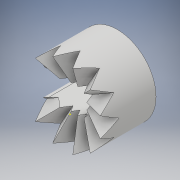
# Autodesk Inventor part: spodek
Saved by Autodesk Inventor 2018 (Build 220112000, 112)
## iProperties
Created: 2017-05-11
Part Number: spodek
Material: Všeobecné
Document SubType Name: Modeling
Designer: tonarr
Density: 1 g/cm^3
Appearance: Výchozí
Author: tonarr
Autodesk Inventor part; units mm, degrees
ref_plane "YZ Plane" through (0, 0, 0) normal (1, 0, 0) x (0, 1, 0)
ref_plane "XZ Plane" through (0, 0, 0) normal (0, 1, 0) x (-1, 0, 0)
sketch "Náčrt1" plane through (0, 0, 0) normal (0, 1, 0) x (-1, 0, 0)
  circle A0 centre (0, 0) radius 12.5
  circle A1 centre (0, 0) radius 2
  circle A2 centre (10, 0) radius 2
  dimension "d0" = 25
  dimension "d1" = 4
  dimension "d2" = 10
  constraints: 3 centre point, 2 coincident, 1 equal radius, 1 horizontal alignment
  measures "d0" diameter of A0
  measures "d1" diameter of A1
  measures "d2" distance of point (0, 0) A2.centre
extrude "Vysunutí1" add sketch "Náčrt1" along normal blind 18
sketch "Náčrt2" plane through (0, 0, 0) normal (1, 0, 0) x (0, 1, 0)
  line L0 (6.0622, 0) -> (0, -3.5)
  line L1 (0, -3.5) -> (0, 3.5)
  line L2 (0, 3.5) -> (6.0622, 0)
  point P0 (0, 0)
  point P1 (2.0207, 0)
  dimension "d5" = 7
  constraints: 6 end point, 1 horizontal alignment, 1 vertical, 1 vertical alignment, 7 other
  measures "d5" distance of L0.end L1.end
extrude "Vysunutí2" cut sketch "Náčrt2" against normal blind 20
pattern_circular "Kruhové pole1" count 12 over 360 about axis through (0, 0, 0) along (0, 1, 0) of "Vysunutí2"
sketch "Náčrt3" plane through (-8.8388, 0.4586, -8.8388) normal (-0.4330127, -0.5, 0.75) x (0.6452387, 0.4090649, 0.6452387)
  point P0 (11.2187, -4.6274)
ref_plane "Pracovní rovina1" through (0, 16, 0) normal (0, 1, 0) x (1, 0, 0)
sketch "Náčrt4" plane through (0, 16, 0) normal (0, 1, 0) x (1, 0, 0)
  line L0 (4, -4) -> (-12.5, -4)
  line L1 (-12.5, -4) -> (-12.5, 4)
  line L2 (-12.5, 4) -> (4, 4)
  line L3 (4, 4) -> (4, -4)
  circle A0 centre (-10, 0) radius 2 projected
  circle A1 centre (0, 0) radius 2 projected
  circle A2 centre (0, 0) radius 12.5 projected
  circle A3 centre (0, 0) radius 12.5 construction
  line L4 (-12.5, 0) -> (-12.5, 13.6221) construction
  point P0 (4, 0)
  dimension "d13" = 8
  dimension "d14" = 16.5
  constraints: 10 end point, 2 horizontal alignment, 2 parallel, 2 vertical, 1 horizontal, 1 midpoint, 1 perpendicular, 1 vertical alignment, 1 other
  measures "d13" distance of L0.end L1.end
  measures "d14" distance of L1.end L2.end
extrude "Vysunutí3" cut sketch "Náčrt4" against normal blind 20 contours L0 A2 L2 L3 | L0 L1 A2 | L1 L2 A2 picked at (-2.8506, -3.29)
fillet "Zaoblení1" radius 2 4 edges at (4, 9.7631, 4) (4, 9.7631, -4) (-11.8427, 8.903, -4) (-11.8427, 8.903, 4)
